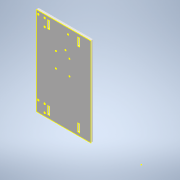
# Autodesk Inventor part: base
Saved by Autodesk Inventor 2022 (Build 260153000, 153)
## iProperties
Created: 2023-05-18
Part Number: base
Material: Типовые
Document SubType Name: Modeling
Designer: Robo0
Density: 1 g/cm^3
Appearance: По умолчанию
Author: Robo0
Autodesk Inventor part; units mm, degrees
ref_plane "YZ Plane" through (0, 0, 0) normal (1, 0, 0) x (0, 1, 0)
ref_plane "XZ Plane" through (0, 0, 0) normal (0, 1, 0) x (-1, 0, 0)
ref_plane "XY Plane" through (0, 0, 0) normal (0, 0, 1) x (1, 0, 0)
sketch "Эскиз1" plane through (0, 0, 0) normal (0, 0, 1) x (1, 0, 0)
  circle A0 centre (-130.7857, -7.8645) radius 2 projected
  circle A1 centre (-146.7857, -7.8645) radius 2 projected
  circle A2 centre (-146.7857, 11.5448) radius 2 projected
  circle A3 centre (-130.7857, 11.5448) radius 2 projected
  circle A4 centre (-257.4369, -7.8494) radius 2 projected
  circle A5 centre (-241.4369, -7.8494) radius 2 projected
  circle A6 centre (-241.4369, 11.5599) radius 2 projected
  circle A7 centre (-257.4369, 11.5599) radius 2 projected
  circle A8 centre (-241.4369, 177.5749) radius 2 projected
  circle A9 centre (-257.4369, 177.5749) radius 2 projected
  circle A10 centre (-241.4369, 196.9843) radius 2 projected
  circle A11 centre (-257.4369, 196.9843) radius 2 projected
  circle A12 centre (-130.7857, 196.9691) radius 2 projected
  circle A13 centre (-130.7857, 177.5598) radius 2 projected
  circle A14 centre (-146.7857, 177.5598) radius 2 projected
  circle A15 centre (-146.7857, 196.9691) radius 2 projected
  line L0 (-126.2857, -20.0509) -> (-126.2857, 23.7311) projected
  line L1 (-11.2, 1) -> (-52.2, 1)
  line L2 (-261.9369, 209.1706) -> (-261.9369, 165.3886) projected
  line L3 (-234.1113, 204.9843) -> (-286.9369, 204.9843) projected
  line L4 (-154.1113, -15.8645) -> (-101.2857, -15.8645) projected
  line L5 (-126.2857, -15.8645) -> (-261.9369, -15.8645)
  line L6 (-261.9369, -15.8645) -> (-261.9369, 204.9843)
  line L7 (-261.9369, 204.9843) -> (-126.2857, 204.9843)
  line L8 (-126.2857, 204.9843) -> (-126.2857, -15.8645)
  point P0 (0, 0)
  point P1 (-261.9369, 209.1706)
  constraints: 10 end point, 4 point on line, 2 horizontal, 2 parallel, 1 perpendicular, 2 other
extrude "Выдавливание1" add sketch "Эскиз1" along normal blind 6 contours A0 | A1 | A2 | A3 | A4 | A5 | A9 | A12 | A13 | A14 | A15 | L4 L5 L6 L2 L3 L7 L8 L0
sketch "Эскиз2" plane through (0, 0, 6) normal (0, 0, 1) x (1, 0, 0)
  circle A0 centre (-183.1113, 190.4843) radius 1.6 projected
  circle A1 centre (-189.4013, 153.4483) radius 1.6 projected
  point P0 (0, 0)
extrude "Выдавливание2" cut sketch "Эскиз2" against normal blind 10
sketch "Эскиз3" plane through (0, 0, 6) normal (0, 0, 1) x (1, 0, 0)
  circle A0 centre (-241.4369, 11.5599) radius 2 projected
  circle A1 centre (-241.4369, -7.8494) radius 2 projected
  line L0 (-234.1113, -15.8645) -> (-234.1113, 19.5599) projected
  line L1 (-234.1113, 11.5599) -> (-229.1113, 11.5599)
  line L2 (-229.1113, 11.5599) -> (-229.1113, -7.8494)
  line L3 (-229.1113, -7.8494) -> (-234.1113, -7.8494)
  line L4 (-234.1113, -7.8494) -> (-234.1113, 11.5599)
  line L5 (-154.1113, 19.5599) -> (-154.1113, -15.8645) projected
  line L6 (-154.1113, 11.5599) -> (-159.1113, 11.5599)
  line L7 (-159.1113, 11.5599) -> (-159.1113, -7.8494)
  line L8 (-159.1113, -7.8494) -> (-154.1113, -7.8494)
  line L9 (-154.1113, -7.8494) -> (-154.1113, 11.5599)
  circle A2 centre (-241.4369, 196.9843) radius 2 projected
  circle A3 centre (-241.4369, 177.5749) radius 2 projected
  line L10 (-234.1113, 196.9843) -> (-229.1113, 196.9843)
  line L11 (-229.1113, 196.9843) -> (-229.1113, 177.5749)
  line L12 (-229.1113, 177.5749) -> (-234.1113, 177.5749)
  line L13 (-234.1113, 177.5749) -> (-234.1113, 196.9843)
  line L14 (-154.1113, 196.9843) -> (-159.1113, 196.9843)
  line L15 (-159.1113, 196.9843) -> (-159.1113, 177.5749)
  line L16 (-159.1113, 177.5749) -> (-154.1113, 177.5749)
  line L17 (-154.1113, 177.5749) -> (-154.1113, 196.9843)
  point P0 (0, 0)
  dimension "d4" = 5
  dimension "d5" = 5
  constraints: 32 end point, 8 parallel, 4 horizontal, 4 perpendicular, 4 point on line
  measures "d4" distance of L2.end L3.end
  measures "d5" distance of L8.end L7.end
extrude "Выдавливание3" cut sketch "Эскиз3" against normal blind 10
sketch "Эскиз4" plane through (0, 0, 6) normal (0, 0, 1) x (1, 0, 0)
  circle A0 centre (-174.157, 139.735) radius 1.5 projected
  circle A1 centre (-207.757, 139.735) radius 1.5 projected
  circle A2 centre (-207.757, 101.735) radius 1.5 projected
  line L0 (-154.1113, 11.5599) -> (-154.1113, -7.8494) projected
  line L1 (-154.1113, -7.8494) -> (-159.1113, -7.8494) projected
  line L2 (-159.1113, -7.8494) -> (-159.1113, 11.5599) projected
  line L3 (-159.1113, 11.5599) -> (-154.1113, 11.5599) projected
  circle A3 centre (-241.4369, -7.8494) radius 2 projected
  line L4 (-234.1113, -7.8494) -> (-234.1113, 11.5599) projected
  line L5 (-234.1113, 11.5599) -> (-229.1113, 11.5599) projected
  line L6 (-229.1113, 11.5599) -> (-229.1113, -7.8494) projected
  line L7 (-229.1113, -7.8494) -> (-234.1113, -7.8494) projected
  line L8 (-229.1113, 196.9843) -> (-229.1113, 177.5749) projected
  line L9 (-229.1113, 177.5749) -> (-234.1113, 177.5749) projected
  line L10 (-234.1113, 177.5749) -> (-234.1113, 196.9843) projected
  line L11 (-234.1113, 196.9843) -> (-229.1113, 196.9843) projected
  line L12 (-154.1113, 177.5749) -> (-159.1113, 177.5749) projected
  line L13 (-159.1113, 177.5749) -> (-159.1113, 196.9843) projected
  line L14 (-159.1113, 196.9843) -> (-154.1113, 196.9843) projected
  line L15 (-154.1113, 196.9843) -> (-154.1113, 177.5749) projected
  circle A4 centre (-183.1113, 190.4843) radius 1.6 projected
  circle A5 centre (-189.4013, 153.4483) radius 1.6 projected
  line L16 (-126.2857, 204.9843) -> (-261.9369, 204.9843) projected
  line L17 (-261.9369, 204.9843) -> (-261.9369, -15.8645) projected
  line L18 (-261.9369, -15.8645) -> (-126.2857, -15.8645) projected
  line L19 (-126.2857, -15.8645) -> (-126.2857, 204.9843) projected
  circle A6 centre (-257.4369, 196.9843) radius 2 projected
  circle A7 centre (-257.4369, 11.5599) radius 2 projected
  circle A8 centre (-241.4369, 11.5599) radius 2 projected
  circle A9 centre (-241.4369, 177.5749) radius 2 projected
  circle A10 centre (-241.4369, 196.9843) radius 2 projected
  circle A11 centre (-174.157, 101.735) radius 1.5 projected
  circle A12 centre (-207.757, 12.735) radius 1.5 projected
  circle A13 centre (-207.757, 50.735) radius 1.5 projected
  circle A14 centre (-174.157, 50.735) radius 1.5 projected
  circle A15 centre (-174.157, 12.735) radius 1.5 projected
  point P0 (0, 0)
extrude "Выдавливание4" cut sketch "Эскиз4" against normal blind 10 contours A0 | A1 | A2 | A11 | A12 | A13 | A14 | A15
sketch "Эскиз5" plane through (0, 0, 6) normal (0, 0, 1) x (1, 0, 0)
  line L0 (-179.457, 56.235) -> (-202.457, 56.235) projected
  line L1 (-202.457, 96.235) -> (-179.457, 96.235) projected
  line L2 (-227.2988, 76.235) -> (-132.8267, 76.235) construction
  line L3 (-222.8708, 67.4513) -> (-222.8708, 191.9683) construction
  line L4 (-227.2988, 168.0107) -> (-230.2988, 168.0107)
  line L5 (-230.2988, 168.0107) -> (-230.2988, 158.0107)
  line L6 (-230.2988, 158.0107) -> (-227.2988, 158.0107)
  line L7 (-227.2988, 158.0107) -> (-227.2988, 168.0107)
  line L8 (-222.8708, 27.4513) -> (-222.8708, 151.9683) construction
  line L9 (-227.2988, 128.0107) -> (-230.2988, 128.0107)
  line L10 (-230.2988, 128.0107) -> (-230.2988, 118.0107)
  line L11 (-230.2988, 118.0107) -> (-227.2988, 118.0107)
  line L12 (-227.2988, 118.0107) -> (-227.2988, 128.0107)
  line L13 (-222.8708, -12.5487) -> (-222.8708, 111.9683) construction
  line L14 (-227.2988, 88.0107) -> (-230.2988, 88.0107)
  line L15 (-230.2988, 88.0107) -> (-230.2988, 78.0107)
  line L16 (-230.2988, 78.0107) -> (-227.2988, 78.0107)
  line L17 (-227.2988, 78.0107) -> (-227.2988, 88.0107)
  line L18 (-214.9907, 78.0107) -> (-204.9907, 78.0107)
  line L19 (-204.9907, 78.0107) -> (-204.9907, 81.0107)
  line L20 (-204.9907, 81.0107) -> (-214.9907, 81.0107)
  line L21 (-214.9907, 81.0107) -> (-214.9907, 78.0107)
  line L22 (-184.9907, 81.0107) -> (-184.9907, 78.0107)
  line L23 (-174.9907, 81.0107) -> (-184.9907, 81.0107)
  line L24 (-184.9907, 78.0107) -> (-174.9907, 78.0107)
  line L25 (-174.9907, 78.0107) -> (-174.9907, 81.0107)
  line L26 (-154.9907, 81.0107) -> (-154.9907, 78.0107)
  line L27 (-144.9907, 81.0107) -> (-154.9907, 81.0107)
  line L28 (-154.9907, 78.0107) -> (-144.9907, 78.0107)
  line L29 (-144.9907, 78.0107) -> (-144.9907, 81.0107)
  line L30 (-218.4428, 168.0107) -> (-215.4428, 168.0107)
  line L31 (-215.4428, 168.0107) -> (-215.4428, 158.0107)
  line L32 (-215.4428, 158.0107) -> (-218.4428, 158.0107)
  line L33 (-218.4428, 158.0107) -> (-218.4428, 168.0107)
  line L34 (-218.4428, 128.0107) -> (-215.4428, 128.0107)
  line L35 (-215.4428, 128.0107) -> (-215.4428, 118.0107)
  line L36 (-215.4428, 118.0107) -> (-218.4428, 118.0107)
  line L37 (-218.4428, 118.0107) -> (-218.4428, 128.0107)
  line L38 (-218.4428, 88.0107) -> (-215.4428, 88.0107)
  line L39 (-215.4428, 88.0107) -> (-215.4428, 78.0107)
  line L40 (-215.4428, 78.0107) -> (-218.4428, 78.0107)
  line L41 (-218.4428, 78.0107) -> (-218.4428, 88.0107)
  line L42 (-214.9907, 74.4594) -> (-204.9907, 74.4594)
  line L43 (-204.9907, 74.4594) -> (-204.9907, 71.4594)
  line L44 (-204.9907, 71.4594) -> (-214.9907, 71.4594)
  line L45 (-184.9907, 71.4594) -> (-184.9907, 74.4594)
  line L46 (-174.9907, 71.4594) -> (-184.9907, 71.4594)
  line L47 (-184.9907, 74.4594) -> (-174.9907, 74.4594)
  line L48 (-174.9907, 74.4594) -> (-174.9907, 71.4594)
  line L49 (-154.9907, 71.4594) -> (-154.9907, 74.4594)
  line L50 (-144.9907, 71.4594) -> (-154.9907, 71.4594)
  line L51 (-154.9907, 74.4594) -> (-144.9907, 74.4594)
  line L52 (-144.9907, 74.4594) -> (-144.9907, 71.4594)
  point P0 (0, 0)
  point P1 (-218.4428, 76.235)
  dimension "d10" = 40
  dimension "d11" = 20
  dimension "d12" = 3
  dimension "d13" = 10
  dimension "d16" = 40
  dimension "d21" = 10
  dimension "d22" = 3
  dimension "d25" = 30
  constraints: 102 end point, 25 symmetric about line, 4 horizontal, 4 parallel, 2 perpendicular, 2 vertical, 1 collinear, 37 other
  measures "d10" distance between parallel lines of L1 L0
  measures "d11" distance between parallel lines of L0 L2
  measures "d12" distance of L6.end L5.end
  measures "d13" distance of L5.end L4.end
  measures "d16" distance of L3.start L8.start
  measures "d21" distance of L20.end L19.end
  measures "d22" distance of L19.end L18.end
  measures "d25" distance of L20.end L22.start
extrude "Выдавливание5" cut sketch "Эскиз5" against normal blind 10
sketch "Эскиз6" plane through (0, 0, 6) normal (0, 0, 1) x (1, 0, 0)
  line L0 (-163.4916, 110.1307) -> (-158.4916, 110.1307)
  line L1 (-158.4916, 110.1307) -> (-158.4916, 107.1307)
  line L2 (-158.4916, 107.1307) -> (-163.4916, 107.1307)
  line L3 (-163.4916, 107.1307) -> (-163.4916, 110.1307)
  line L4 (-143.4916, 110.1307) -> (-138.4916, 110.1307)
  line L5 (-138.4916, 110.1307) -> (-138.4916, 107.1307)
  line L6 (-138.4916, 107.1307) -> (-143.4916, 107.1307)
  line L7 (-143.4916, 107.1307) -> (-143.4916, 110.1307)
  line L8 (-168.9534, 113.1307) -> (-129.2499, 113.1307) construction
  line L9 (-163.4916, 116.1307) -> (-158.4916, 116.1307)
  line L10 (-158.4916, 116.1307) -> (-158.4916, 119.1307)
  line L11 (-158.4916, 119.1307) -> (-163.4916, 119.1307)
  line L12 (-163.4916, 119.1307) -> (-163.4916, 116.1307)
  line L13 (-143.4916, 116.1307) -> (-138.4916, 116.1307)
  line L14 (-138.4916, 116.1307) -> (-138.4916, 119.1307)
  line L15 (-138.4916, 119.1307) -> (-143.4916, 119.1307)
  line L16 (-143.4916, 119.1307) -> (-143.4916, 116.1307)
  line L17 (-165.5611, 35.1192) -> (-160.5611, 35.1192)
  line L18 (-160.5611, 35.1192) -> (-160.5611, 32.1192)
  line L19 (-160.5611, 32.1192) -> (-165.5611, 32.1192)
  line L20 (-165.5611, 32.1192) -> (-165.5611, 35.1192)
  line L21 (-145.5611, 35.1192) -> (-140.5611, 35.1192)
  line L22 (-140.5611, 35.1192) -> (-140.5611, 32.1192)
  line L23 (-140.5611, 32.1192) -> (-145.5611, 32.1192)
  line L24 (-145.5611, 32.1192) -> (-145.5611, 35.1192)
  line L25 (-165.5611, 41.1192) -> (-160.5611, 41.1192)
  line L26 (-160.5611, 41.1192) -> (-160.5611, 44.1192)
  line L27 (-160.5611, 44.1192) -> (-165.5611, 44.1192)
  line L28 (-165.5611, 44.1192) -> (-165.5611, 41.1192)
  line L29 (-145.5611, 41.1192) -> (-140.5611, 41.1192)
  line L30 (-140.5611, 41.1192) -> (-140.5611, 44.1192)
  line L31 (-140.5611, 44.1192) -> (-145.5611, 44.1192)
  line L32 (-145.5611, 44.1192) -> (-145.5611, 41.1192)
  line L33 (-239.8485, 107.703) -> (-234.8485, 107.703)
  line L34 (-234.8485, 107.703) -> (-234.8485, 104.703)
  line L35 (-234.8485, 104.703) -> (-239.8485, 104.703)
  line L36 (-239.8485, 104.703) -> (-239.8485, 107.703)
  line L37 (-219.8485, 107.703) -> (-214.8485, 107.703)
  line L38 (-214.8485, 107.703) -> (-214.8485, 104.703)
  line L39 (-214.8485, 104.703) -> (-219.8485, 104.703)
  line L40 (-219.8485, 104.703) -> (-219.8485, 107.703)
  line L41 (-239.8485, 113.703) -> (-234.8485, 113.703)
  line L42 (-234.8485, 113.703) -> (-234.8485, 116.703)
  line L43 (-234.8485, 116.703) -> (-239.8485, 116.703)
  line L44 (-239.8485, 116.703) -> (-239.8485, 113.703)
  line L45 (-219.8485, 113.703) -> (-214.8485, 113.703)
  line L46 (-214.8485, 113.703) -> (-214.8485, 116.703)
  line L47 (-214.8485, 116.703) -> (-219.8485, 116.703)
  line L48 (-219.8485, 116.703) -> (-219.8485, 113.703)
  line L49 (-236.918, 32.6914) -> (-236.918, 29.6914)
  line L50 (-236.918, 38.6914) -> (-236.918, 41.6914)
  line L51 (-241.918, 32.6914) -> (-236.918, 32.6914)
  line L52 (-236.918, 29.6914) -> (-241.918, 29.6914)
  line L53 (-241.918, 38.6914) -> (-236.918, 38.6914)
  line L54 (-236.918, 41.6914) -> (-241.918, 41.6914)
  line L55 (-241.918, 41.6914) -> (-241.918, 38.6914)
  line L56 (-241.918, 29.6914) -> (-241.918, 32.6914)
  line L57 (-221.918, 29.6914) -> (-221.918, 32.6914)
  line L58 (-221.918, 41.6914) -> (-221.918, 38.6914)
  line L59 (-216.918, 29.6914) -> (-221.918, 29.6914)
  line L60 (-221.918, 32.6914) -> (-216.918, 32.6914)
  line L61 (-221.918, 38.6914) -> (-216.918, 38.6914)
  line L62 (-216.918, 41.6914) -> (-221.918, 41.6914)
  line L63 (-216.918, 32.6914) -> (-216.918, 29.6914)
  line L64 (-216.918, 38.6914) -> (-216.918, 41.6914)
  point P0 (0, 0)
  point P1 (-245.3103, 110.703)
  dimension "d32" = 3
  dimension "d33" = 5
  dimension "d36" = 20
  dimension "d41" = 3
  dimension "d42" = 3
  dimension "d47" = 3
  dimension "d48" = 5
  dimension "d49" = 20
  dimension "d59" = 3
  dimension "d60" = 5
  dimension "d61" = 20
  dimension "d62" = 3
  dimension "d63" = 5
  dimension "d64" = 20
  constraints: 130 end point, 9 horizontal, 8 parallel, 4 collinear, 4 perpendicular, 28 other
  measures "d32" distance of L2.end L0.start
  measures "d33" distance of L1.end L2.end
  measures "d36" distance of L0.start L4.start
  measures "d41" distance between parallel lines of L0 L8
  measures "d42" distance between parallel lines of L8 L9
  measures "d47" distance of L19.end L17.start
  measures "d48" distance of L18.end L19.end
  measures "d49" distance of L17.start L24.end
  measures "d59" distance of L35.end L33.start
  measures "d60" distance of L34.end L35.end
  measures "d61" distance of L33.start L40.end
  measures "d62" distance of L52.end L56.end
  measures "d63" distance of L49.end L52.end
  measures "d64" distance of L56.end L60.start
extrude "Выдавливание6" cut sketch "Эскиз6" against normal blind 10
